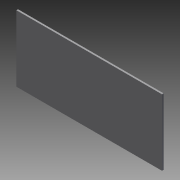
# Autodesk Inventor part: electrical board front top
Saved by Autodesk Inventor 2012 (Build 160160000, 160)
## iProperties
Created: 2012-01-14
Part Number: electrical board front top
Material: ABS Plastic
Document SubType Name: Modeling
Designer: Antonella Wilby
Density: 1.06 g/cm^3
Mass: 1250.66 g
Surface Area: 3832.25 cm^2
Volume: 1179.87 cm^3
Author: Antonella Wilby
Autodesk Inventor part; units mm, degrees
ref_plane "YZ Plane" through (0, 0, 0) normal (1, 0, 0) x (0, 1, 0)
ref_plane "XZ Plane" through (0, 0, 0) normal (0, 1, 0) x (-1, 0, 0)
ref_plane "XY Plane" through (0, 0, 0) normal (0, 0, 1) x (1, 0, 0)
sketch "Sketch1" plane through (0, 0, 0) normal (0, 0, 1) x (1, 0, 0)
  line L0 (-391.16, 0) -> (391.16, 0) projected
  line L1 (0, -177.8) -> (0, 177.8) projected
  line L2 (-279.4, 127) -> (279.4, 127)
  line L3 (279.4, 127) -> (279.4, -127)
  line L4 (279.4, -127) -> (-279.4, -127)
  line L5 (-279.4, -127) -> (-279.4, 127)
  point P0 (0, 0)
  point P1 (-279.4, 0)
  point P2 (0, 127)
  dimension "d0" = 558.8
  dimension "d1" = 254
  constraints: 8 end point, 2 midpoint, 2 parallel, 1 horizontal, 1 horizontal alignment, 1 perpendicular, 1 vertical alignment
  measures "d0" distance of L2.start L2.end
  measures "d1" distance of L4.end L2.start
extrude "Extrusion1" add sketch "Sketch1" along normal mid plane 6.35
body "Solid1"
